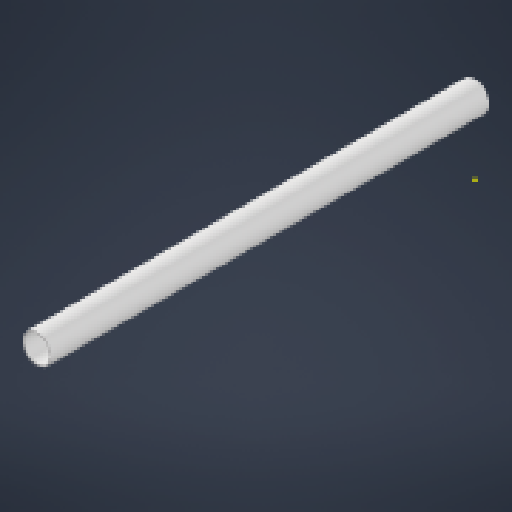
# Autodesk Inventor part: wal
Saved by Autodesk Inventor 2025 (Build 290162000, 162)
## iProperties
Created: 2024-04-14
Part Number: wal
Material: Generic
Document SubType Name: Modeling
Designer: sicia
Density: 1 g/cm^3
Appearance: Default
Author: sicia
Autodesk Inventor part; units mm, degrees
ref_plane "YZ Plane" through (0, 0, 0) normal (1, 0, 0) x (0, 1, 0)
ref_plane "XZ Plane" through (0, 0, 0) normal (0, 1, 0) x (-1, 0, 0)
ref_plane "XY Plane" through (0, 0, 0) normal (0, 0, 1) x (1, 0, 0)
sketch "Sketch1" plane through (0, 0, 0) normal (0, 0, 1) x (1, 0, 0)
  circle A0 centre (0, 50) radius 18.5 projected
  circle A1 centre (0, 50) radius 18.5 projected
  circle A2 centre (0, 50) radius 18.5 projected
  circle A3 centre (0, 50) radius 21.5 projected
  circle A4 centre (0, 50) radius 18.5 projected
  circle A5 centre (0, 50) radius 10
  circle A6 centre (0, 50) radius 9
  point P0 (0, 0)
  dimension "d0" = 20
  dimension "d5" = 18
  constraints: 2 centre point, 2 coincident
  measures "d0" diameter of A5
  measures "d5" diameter of A6
extrude "Extrusion1" add sketch "Sketch1" along normal blind 50 and the other way blind 250 contours A5
sketch "Sketch2" plane through (0, 50, -250) normal (0, 0, -1) x (-1, 0, 0)
  point P0 (0, -50)
body "Solid1"
